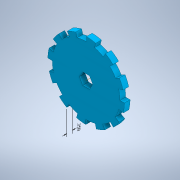
# Autodesk Inventor part: gearLock
Saved by Autodesk Inventor 2022.1 (Build 261234000, 234)
## iProperties
Created: 2020-11-07
Part Number: gearLock
Material: PC/ABS Plastic
Document SubType Name: Modeling
Designer: robst
Density: 0.357273 g/cm^3
Appearance: Sky Blue Medium
Author: robst
Autodesk Inventor part; units mm, degrees
ref_plane "YZ Plane" through (0, 0, 0) normal (1, 0, 0) x (0, 1, 0)
ref_plane "XZ Plane" through (0, 0, 0) normal (0, 1, 0) x (-1, 0, 0)
ref_plane "XY Plane" through (0, 0, 0) normal (0, 0, 1) x (1, 0, 0)
sketch "Sketch1" plane through (0, 0, 0) normal (0, 0, 1) x (1, 0, 0)
  circle A0 centre (0, 0) radius 37.9095
  dimension "d0" = 75.819
  constraints: 1 centre point, 1 coincident
  measures "d0" diameter of A0
extrude "Extrusion1" add sketch "Sketch1" along normal mid plane 6.35
sketch "Sketch10" plane through (0, 0, 3.175) normal (0, 0, 1) x (1, 0, 0)
  line L0 (7.5523, 0) -> (3.7762, -6.5405)
  line L1 (3.7762, -6.5405) -> (-3.7762, -6.5405)
  line L2 (-3.7762, -6.5405) -> (-7.5523, 0)
  line L3 (-7.5523, 0) -> (-3.7762, 6.5405)
  line L4 (-3.7762, 6.5405) -> (3.7762, 6.5405)
  line L5 (3.7762, 6.5405) -> (7.5523, 0)
  point P0 (0, 0)
  point P1 (0, 0)
  dimension "d55" = 13.081
  constraints: 12 end point, 1 coincident, 1 horizontal, 13 other
  measures "d55" distance between parallel lines of L1 L4
extrude "Extrusion11" cut sketch "Sketch10" against normal through all
sketch "Sketch17" plane through (0, 0, 3.175) normal (0, 0, 1) x (1, 0, 0)
  circle A0 centre (0, 0) radius 37.9095 projected
  arc A1 (9.4918, 36.702) -> (0, 37.9095) centre (0, 0) ccw
  arc A2 (10.7405, 41.5304) -> (0, 42.8968) centre (0, 0) ccw
  line L0 (0, 0) -> (0, 42.8968) construction
  line L1 (0, 0) -> (0.3743, 42.8951)
  line L2 (9.4918, 36.702) -> (10.7405, 41.5304)
  point P0 (0.3308, 37.9081)
  dimension "d123" = 4.9873
  dimension "d124" = 0.5
  dimension "d125" = 14
  dimension "d131" = 75.819
  dimension "d132" = 85.7936
  constraints: 6 end point, 5 point on circle, 2 centre point, 2 coincident, 1 concentric, 1 point on line, 1 vertical
  measures "d123" radial gap between concentric circles of A2 A0
  measures "d124" angle of L1 L0
  measures "d125" angle of L2 L1
  measures "d131" diameter of A0
  measures "d132" diameter of A2
extrude "Extrusion19" add sketch "Sketch17" against normal blind 6.35 contours A0 L1 A2 L2
pattern_circular "Circular Pattern11" count 12 over 360 about axis through (0, 0, -10) along (0, 0, 1) of "Extrusion19"
equation "\"d0\" = externalDiameter - 2 * printSpacing"
equation "\"d55\" = hexSize + 2 * printSpacing"
equation "\"d123\" = depthOfExternalSpline"
equation "\"d124\" = 0.5 * absPrintSpacingAngleDiff"
equation "\"d125\" = angleForSplineTooth"
equation "\"d126\" = thickness"
equation "\"internalDiameter\" = 50.8"
equation "\"externalDiameter\" = 76.2"
equation "\"pi\" = 3.141593"
equation "\"depthOfInternalSpline\" = 0.5 * widthOfInternalSpline"
equation "\"thickness\" = 6.35"
equation "\"hexSize\" = 12.7"
equation "\"printSpacing\" = 0.1905"
equation "\"holeDiameterForBushing\" = 50.8"
equation "\"printSpacingAngleDiff\" = -1deg"
equation "\"gapSpacing\" = 7.9375"
equation "\"oneHalfGapSpacing\" = 0.5 * gapSpacing"
equation "\"gapDepth\" = 7.14375"
equation "\"gapCircleDiameter\" = 63.5"
equation "\"shouldBoltSpaceing\" = 4.7625"
equation "\"oneHalfShouldBoltSpacing\" = 0.5 * shouldBoltSpaceing"
equation "\"shoulderBoltDiameter\" = 4.7625"
equation "\"shoulderBoltHeadDiameter\" = 7.9375"
equation "\"shoulderBoltHeadSize\" = 3.96875"
equation "\"depthOfExternalSpline\" = 4.987278"
equation "\"absPrintSpacingAngleDiff\" = 1deg"
equation "\"angleForSplineTooth\" = 14deg"
equation "\"widthOfInternalSpline\" = 6.649704"
body "Solid1"
